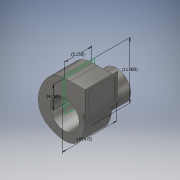
# Autodesk Inventor part: dayton1TDT2 $167
Saved by Autodesk Inventor 2017 (Build 210142000, 142)
## iProperties
Created: 2019-04-12
Part Number: dayton1TDT2 $167
Material: Steel, Mild
Document SubType Name: Modeling
Designer: Brian
Density: 7.85 g/cm^3
Appearance: Semi-Polished
Author: Brian
spiral_factor: 1.160 ul
Autodesk Inventor part; units mm, degrees
ref_plane "YZ Plane" through (0, 0, 0) normal (1, 0, 0) x (0, 1, 0)
ref_plane "XZ Plane" through (0, 0, 0) normal (0, 1, 0) x (-1, 0, 0)
ref_plane "XY Plane" through (0, 0, 0) normal (0, 0, 1) x (1, 0, 0)
sketch "Sketch1" plane through (0, 0, 0) normal (0, 0, 1) x (1, 0, 0)
  circle A0 centre (0, 0) radius 71.0197
  circle A1 centre (0, 0) radius 83.5526 construction
  line L0 (112.4284, 154.4541) -> (112.4284, 46.5041)
  line L1 (112.4284, 154.4541) -> (27.2344, 154.4541)
  line L2 (0, 0) -> (0, 151.2837) construction
  arc A2 (-130.2928, 5.6887) -> (-130.2928, -5.6887) centre (0, 0) ccw
  line L3 (0, 0) -> (-130.2928, 5.6887) construction
  line L4 (0, 0) -> (-130.2928, -5.6887) construction
  arc A3 (-4.9041, -112.3214) -> (4.9041, -112.3214) centre (0, 0) ccw
  line L5 (0, 0) -> (4.9041, -112.3214) construction
  line L6 (0, 0) -> (-4.9041, -112.3214) construction
  spline S0 degree 4 poles (-130.2928, -5.6887) (-129.252, -29.5283) (-115.5385, -76.6996) (-72.5309, -97.0894) (-27.6247, -111.3294) (-4.9041, -112.3214) knots 0 0 0 0 0 0.5 1 1 1 1 1
  arc A4 (96.9211, 0) -> (91.076, 33.149) centre (0, 0) ccw
  line L7 (0, 0) -> (91.076, 33.149) construction
  spline S1 degree 4 poles (96.9211, 0) (96.9211, -20.205) (85.6887, -60.6151) (67.8997, -98.9275) (26.0572, -111.3978) (4.9041, -112.3214) knots 0 0 0 0 0 0.5 1 1 1 1 1
  line L8 (112.4284, 46.5041) -> (99.7284, 46.5041)
  spline S2 degree 4 poles (99.7284, 46.5041) (97.2855, 46.5041) (92.3997, 46.5041) (88.4826, 39.817) (90.2605, 35.3895) (91.076, 33.149) knots 0 0 0 0 0 0.5 1 1 1 1 1
  line L9 (0, 0) -> (0, -253.3414) construction
  line L10 (0, 0) -> (-251.0409, 0) construction
  line L11 (0, 0) -> (96.9211, 0) construction
  line L12 (112.4284, 154.4541) -> (112.4284, 167.1541)
  line L13 (112.4284, 72.3116) -> (112.4284, 0) construction
  line L14 (0, 0) -> (27.2344, 154.4541) construction
  spline S3 degree 4 poles (27.2344, 154.4541) (-3.5458, 154.4541) (-65.1062, 154.4541) (-106.7346, 97.4701) (-128.9447, 36.5665) (-130.2928, 5.6887) knots 0 0 0 0 0 0.5 1 1 1 1 1
  line L15 (96.9211, 0) -> (112.4284, 0) construction
  line L16 (99.7284, 46.5041) -> (0, 0) construction
  line L17 (112.4284, 46.5041) -> (112.4284, 33.8041)
  line L18 (0, -112.4284) -> (163.7102, -112.4284) construction
  line L19 (112.4284, 167.1541) -> (187.2501, 167.1541) construction
  line L20 (-130.417, 0) -> (-130.417, 167.1541) construction
  line L21 (-130.417, 167.1541) -> (112.4284, 167.1541) construction
  dimension "inlet_radius" = 71.0197
  dimension "blower_wheel_radius" = 83.5526
  dimension "outlet_height" = 107.95
  dimension "d8" = 151.2837
  dimension "d13" = 130.417
  dimension "d15" = 5
  dimension "d16" = 112.4284
  dimension "d18" = 5
  dimension "d19" = 90
  dimension "d20" = 96.921
  dimension "d24" = 12.7
  dimension "d25" = 112.4284
  dimension "d26" = 12.7
  dimension "d28" = 10
  dimension "d29" = 20
  dimension "d32" = 25
  dimension "d33" = 12.7
  dimension "d39" = 279.5826
  dimension "d40" = 242.8454
  constraints: 44 end point, 8 point on circle, 6 coincident, 6 horizontal, 6 vertical, 5 centre point, 3 perpendicular, 3 point on line, 1 collinear, 14 other
  measures "inlet_radius" radius of A0
  measures "blower_wheel_radius" radius of A1
  measures "outlet_height" distance of L0.end L0.start
  measures "d8" distance of L2.start L2.end
  measures "d13" radius of A2
  measures "d15" angle of L3 L4
  measures "d16" radius of A3
  measures "d18" angle of L6 L5
  measures "d19" angle of L1 L2
  measures "d20" radius of A4
  measures "d24" distance of L0.end L8.end
  measures "d25" distance of L7.start L13.end
  measures "d26" distance of L0.start L12.end
  measures "d28" angle of L14 L2
  measures "d29" angle of L11 L7
  measures "d32" angle of L11 L16
  measures "d33" distance of L0.end L17.end
  measures "d39" distance between parallel lines of L19 L18
  measures "d40" distance of L20.end L12.end
extrude "Extrusion1" add sketch "Sketch1" along normal blind 133.35
sketch "Sketch2" plane through (112.4284, 46.5041, 0) normal (1, 0, 0) x (0, 0, -1)
  line L0 (0, 107.95) -> (0, 0) projected
  line L1 (0, 107.95) -> (-133.35, 107.95) projected
  line L2 (-133.35, 0) -> (-133.35, 107.95) projected
  line L3 (0, 0) -> (-133.35, 0) projected
  line L4 (-146.05, 120.65) -> (12.7, 120.65)
  line L5 (12.7, 120.65) -> (12.7, -12.7)
  line L6 (12.7, -12.7) -> (-146.05, -12.7)
  line L7 (-146.05, -12.7) -> (-146.05, 120.65)
  point P0 (0, -46.5041)
  dimension "d34" = 12.7
  constraints: 8 end point, 3 other
  measures "d34" distance between parallel lines of L1 L4
extrude "Extrusion2" add sketch "Sketch2" along normal blind 2.54
extrude "Extrusion3" add sketch "Sketch1" against normal blind 120.015 contours A0
sketch "Sketch3" plane through (0, 0, 0) normal (1, 0, 0) x (0, 1, 0)
  line L0 (33.149, 133.35) -> (46.5041, 133.35) projected
  line L1 (46.5041, 0) -> (46.5041, 133.35) projected
  line L2 (46.5041, 133.35) -> (154.4541, 133.35) projected
  line L3 (154.4541, 133.35) -> (154.4541, 0) projected
  line L4 (154.4541, 0) -> (46.5041, 0) projected
  line L5 (167.1541, -12.7) -> (167.1541, 146.05) projected
  line L6 (167.1541, 146.05) -> (33.8041, 146.05) projected
  line L7 (33.8041, 146.05) -> (33.8041, -12.7) projected
  line L8 (33.8041, -12.7) -> (167.1541, -12.7) projected
  line L9 (33.149, 0) -> (0, 0) projected
  line L10 (33.149, 0) -> (33.149, 133.35) projected
  line L11 (0, 133.35) -> (33.149, 133.35) projected
  line L12 (0, 0) -> (0, 133.35) projected
  line L13 (-71.0197, -120.015) -> (71.0197, -120.015) projected
  line L14 (71.0197, 0) -> (-71.0197, 0) projected
  line L15 (-112.3214, 0) -> (-112.3214, 133.35) projected
  point P0 (0, 0)
  dimension "d41" = 133.35
  dimension "d42" = 107.95
  dimension "d43" = 266.065
  dimension "d44" = 279.4755
  measures "d41" distance between parallel lines of L4 L2
  measures "d42" distance between parallel lines of L1 L3
  measures "d43" distance between parallel lines of L13 L6
  measures "d44" distance between parallel lines of L15 L5
equation "\"d33\" = d26"
equation "\"d37\" = 0.9 * outlet_width"
equation "\"spiral_factor\" = 1.16"
equation "\"blower_wheel_width\" = 80.9625"
equation "\"outlet_width\" = 133.35"
body "Solid1"
